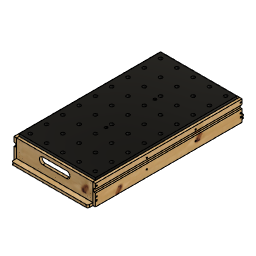
Make_Werkbank v11 (Autodesk Fusion 360 design; units mm, degrees)
Autodesk Fusion 360 part; units mm, degrees
note: some values were not read from the file. Set by a fixed rule: which face or edge a step refers to.
sketch "Seite_L" plane through (0, 0, 0) normal (1, 0, 0) x (0, 1, 0)
  line L0 (432, 60) -> (-432, 60)
  line L1 (-432, 60) -> (-432, -60)
  line L2 (-432, -60) -> (432, -60)
  line L3 (432, -60) -> (432, 60)
  line L4 (432, 60) -> (-432, -60) construction
  line L5 (-432, 60) -> (432, -60) construction
  line L6 (432, 30) -> (-432, 30)
  line L7 (-432, 30) -> (-432, 10)
  line L8 (-432, 10) -> (432, 10)
  line L9 (432, 10) -> (432, 30)
  line L10 (-424.5, -60) -> (-424.5, 60) construction
  line L11 (424.5, -60) -> (424.5, 60) construction
  circle A0 centre (-424.5, 45) radius 4
  circle A1 centre (-424.5, -30) radius 4
  circle A2 centre (-424.5, -10) radius 4
  line L12 (0, -60) -> (0, 60) construction
  circle A3 centre (424.5, 45) radius 4
  circle A4 centre (424.5, -30) radius 4
  circle A5 centre (424.5, -10) radius 4
  point P0 (424.5, 60)
  dimension "d10" = 864
  dimension "d11" = 120
  dimension "d58" = 864
  dimension "d59" = 20
  dimension "d65" = 30
  dimension "d67" = 7.5
  dimension "d68" = 7.5
  dimension "d70" = 8
  dimension "d71" = 15
  dimension "d72" = 8
  dimension "d73" = 8
  dimension "d74" = 30
  dimension "d75" = 20
  constraint horizontal L0
  constraint perpendicular L0 L1
  constraint parallel L1 L3
  constraint coincident L4 origin
  constraint coincident L5 origin
  constraint horizontal L6
  constraint vertical L7
  constraint horizontal L8
  constraint vertical L9
  constraint coincident L3 L6.start
  constraint coincident L2 L10.start
  constraint coincident L0 L10.end
  constraint perpendicular L0 L10
  constraint coincident L2 L11.start
  constraint coincident L0 P0
  constraint perpendicular L0 L11
  constraint coincident L10 A0.centre
  constraint coincident L10 A1.centre
  constraint coincident L10 A2.centre
  constraint midpoint L2 L12.start
  constraint midpoint L0 L12.end
  constraint symmetric L10.end L12 P0
  constraint symmetric A0 L12 A3
  constraint symmetric A1 L12 A4
  constraint symmetric A2 L12 A5
  measures "d10" distance of L1.end L2.end
  measures "d11" distance of L0.end L1.end
  measures "d58" distance of L6.start L6.end
  measures "d59" distance of L6.start L8.end
  measures "d65" distance of L0 L6
  measures "d67" distance of L1 L10
  measures "d68" distance of L3 L11
  measures "d70" diameter of A0
  measures "d71" distance of L0 A0.centre
  measures "d72" diameter of A1
  measures "d73" diameter of A2
  measures "d74" distance of L2 A1.centre
  measures "d75" distance of A1.centre A2.centre
extrude "Extrude1" add sketch "Seite_L" along normal blind 15 contours L0 L1 L3 L6 | L1 L3 L6 L7 L8 L9 | L1 L2 L3 L8 | A0 | A1 | A2 | A3 | A4 | A5 makes body 1
copy_body "CopyPasteBodies2" bodies 1 makes body 2
move_body "Move2" bodies 2 to x (1, 0, 0) y (0, 1, 0) z (0, 0, 1) at (465, 0, 0)
sketch "Seite_K" plane through (0, 0, 0) normal (0, 1, 0) x (1, 0, 0)
  line L0 (15, 45) -> (465, 45)
  line L1 (465, 45) -> (465, -60)
  line L2 (465, -60) -> (15, -60)
  line L3 (15, -60) -> (15, 45)
  line L4 (15, 45) -> (465, 45)
  line L5 (465, 45) -> (465, -55)
  line L6 (465, -55) -> (15, -55)
  line L7 (15, -55) -> (15, 45)
  line L8 (240, -55) -> (240, 45) construction
  line L9 (310, 0) -> (170, 0)
  arc A0 (170, 0) -> (170, -40) centre (170, -20) ccw
  line L10 (170, -40) -> (310, -40)
  arc A1 (310, -40) -> (310, 0) centre (310, -20) ccw
  line L11 (310, -20) -> (170, -20) construction
  line L12 (465, -55) -> (15, -55)
  line L13 (15, -55) -> (15, -40)
  line L14 (15, -40) -> (465, -40)
  line L15 (465, -40) -> (465, -55)
  line L16 (465, -47.5) -> (15, -47.5) construction
  circle A2 centre (432, -47.5) radius 4
  circle A3 centre (336, -47.5) radius 4
  circle A4 centre (240, -47.5) radius 4
  circle A5 centre (144, -47.5) radius 4
  circle A6 centre (48, -47.5) radius 4
  line L17 (465, -60) -> (15, -60)
  line L18 (15, -60) -> (15, -79) construction
  line L19 (15, -79) -> (465, -79) construction
  line L20 (465, -79) -> (465, -60) construction
  circle A7 centre (240, -22) radius 6
  point P0 (240, -20)
  dimension "d16" = 450
  dimension "d17" = 105
  dimension "d28" = 100
  dimension "d54" = 70
  dimension "d55" = 40
  dimension "d96" = 450
  dimension "d97" = 15
  dimension "d98" = 8
  dimension "d99" = 33
  dimension "d103" = 0
  dimension "d144" = 450
  dimension "d145" = 19
  dimension "d146" = 12
  dimension "d155" = 57
  constraint horizontal L0
  constraint vertical L1
  constraint horizontal L2
  constraint vertical L3
  constraint horizontal L4
  constraint vertical L5
  constraint horizontal L6
  constraint vertical L7
  constraint midpoint L6 L8.start
  constraint midpoint L0 L8.end
  constraint perpendicular L0 L8
  constraint tangent L9 A0
  constraint tangent A0 L10
  constraint parallel L9 L10
  constraint tangent L10 A1
  constraint tangent L9 A1
  constraint perpendicular L8 L11
  constraint coincident L8 P0
  constraint midpoint L11 P0
  constraint horizontal L12
  constraint vertical L13
  constraint horizontal L14
  constraint vertical L15
  constraint midpoint L15 L16.start
  constraint midpoint L13 L16.end
  constraint coincident L16 A2.centre
  constraint collinear L10 L14
  constraint horizontal L17
  constraint vertical L18
  constraint horizontal L19
  constraint vertical L20
  constraint coincident L8 A7.centre
  measures "d16" distance of L0.start L0.end
  measures "d17" distance of L0.start L2.end
  measures "d28" distance of L0.start L6.end
  measures "d54" distance of A0.centre P0
  measures "d55" diameter of A0
  measures "d96" distance of L5.end L6.end
  measures "d97" distance of L5.end L14.end
  measures "d98" diameter of A2
  measures "d99" distance of L5 A2.centre
  measures "d144" distance of L1.end L2.end
  measures "d145" distance of L1.end L19.end
  measures "d146" diameter of A7
  measures "d155" distance of L19 A7.centre
extrude "Extrude2" add sketch "Seite_K" against normal blind 15 from surface at 432 separate body contours L0 L1 L3 L4 L5 L7 L9 A0 A1 L14 | L1 L3 L5 L6 L7 L10 L12 L13 L14 L15 | L1 L2 L3 L6 L12 L17 | A2 | A3 | A4 | A5 | A6 makes body 3
copy_body "CopyPasteBodies3" bodies 3 makes body 4
move_body "Move3" bodies 4 to x (1, 0, 0) y (0, 1, 0) z (0, 0, 1) at (0, -849, 0)
sketch "Top" plane through (0, 0, 60) normal (0, 0, 1) x (-1, 0, 0)
  line L0 (-465, 417) -> (-15, 417)
  line L1 (-15, 417) -> (-15, 432)
  line L2 (-15, 432) -> (-465, 432)
  line L3 (-465, 432) -> (-465, 417)
  line L4 (-465, 417) -> (-15, 417)
  line L5 (-15, 417) -> (-15, -417)
  line L6 (-15, -417) -> (-465, -417)
  line L7 (-465, -417) -> (-465, 417)
  line L8 (-15, 417) -> (-465, 417)
  line L9 (-465, 417) -> (-465, 432)
  line L10 (-465, 432) -> (-15, 432)
  line L11 (-15, 432) -> (-15, 417)
  line L12 (-15, 424.5) -> (-465, 424.5) construction
  circle A0 centre (-48, 424.5) radius 4
  line L13 (0, 432) -> (0, -432)
  circle A1 centre (-144, 424.5) radius 4
  circle A2 centre (-240, 424.5) radius 4
  circle A3 centre (-336, 424.5) radius 4
  circle A4 centre (-432, 424.5) radius 4
  line L14 (-15, 0) -> (-465, 0) construction
  circle A5 centre (-336, -424.5) radius 4
  circle A6 centre (-144, -424.5) radius 4
  circle A7 centre (-48, -424.5) radius 4
  circle A8 centre (-240, -424.5) radius 4
  circle A9 centre (-432, -424.5) radius 4
  line L15 (-465, 129) -> (-15, 129) construction
  line L16 (-465, -159) -> (-465.0582, -159)
  line L17 (-465.0582, -159) -> (-15, -159) construction
  circle A10 centre (-240, 129) radius 4
  circle A11 centre (-240, 129) radius 8
  circle A12 centre (-240.0291, -159) radius 4
  circle A13 centre (-240.0291, -159) radius 8
  line L18 (-240, 417) -> (-240, -417) construction
  dimension "d24" = 450
  dimension "d25" = 834
  dimension "d83" = 8
  dimension "d84" = 48
  dimension "d88" = 0
  dimension "d134" = 288
  dimension "d135" = 288
  dimension "d136" = 8
  dimension "d141" = 16
  dimension "d142" = 8
  dimension "d143" = 16
  constraint horizontal L4
  constraint vertical L5
  constraint horizontal L6
  constraint vertical L7
  constraint coincident L0.start L3.end
  constraint horizontal L8
  constraint vertical L9
  constraint horizontal L10
  constraint vertical L11
  constraint coincident L2.end L3.start
  constraint coincident L0.end L1.start
  constraint midpoint L11 L12.start
  constraint midpoint L9 L12.end
  constraint coincident L12 A0.centre
  constraint midpoint L5 L14.start
  constraint midpoint L7 L14.end
  constraint symmetric A0 L14 A7
  constraint symmetric A1 L14 A6
  constraint symmetric A2 L14 A8
  constraint symmetric A3 L14 A5
  constraint symmetric A4 L14 A9
  constraint coincident L7 L15.start
  constraint coincident L5 L15.end
  constraint perpendicular L5 L15
  constraint coincident L7 L16.start
  constraint perpendicular L7 L16
  constraint coincident L5 L17.end
  constraint perpendicular L5 L17
  constraint midpoint L15 A10.centre
  constraint concentric A10 A11
  constraint midpoint L17 A12.centre
  constraint concentric A12 A13
  constraint midpoint L8 L18.start
  constraint midpoint L6 L18.end
  measures "d24" distance of L0.start L0.end
  measures "d25" distance of L0.start L6.end
  measures "d83" diameter of A0
  measures "d84" distance of A0.centre L13
  measures "d134" distance of L4 L15
  measures "d135" distance of L15 L17
  measures "d136" diameter of A10
  measures "d141" diameter of A11
  measures "d142" diameter of A12
  measures "d143" diameter of A13
extrude "Extrude3" add sketch "Top" along normal blind 19 separate body contours L0 L4 L5 L6 L7 L8 | A10 | A11 | A12 | A13 makes body 5
extrude "Extrude4" add sketch "Seite_K" along normal blind 15 from surface at 151.5 separate body contours L0 L1 L3 L4 L5 L7 L9 A0 A1 L14 | L1 L3 L5 L6 L7 L10 L12 L13 L14 L15 | L9 A0 L10 A1 L14 | A2 | A3 | A4 | A5 | A6 | A7 makes body 6
copy_body "CopyPasteBodies4" bodies 6 makes body 7
move_body "Move4" bodies 7 to x (1, 0, 0) y (0, 1, 0) z (0, 0, 1) at (0, -288, 0)
move_body "Align1" bodies 5 to x (1, 0, 0) y (0, 1, 0) z (0, 0, 1) at (0, 0, -5)
sketch "Fuss" plane through (0, 0, -45) normal (0, 0, -1) x (1, 0, 0)
  line L0 (15, 417) -> (465, 417)
  line L1 (465, 417) -> (465, 432)
  line L2 (465, 432) -> (15, 432)
  line L3 (15, 432) -> (15, 417)
  line L4 (15, 417) -> (465, 417)
  line L5 (465, 417) -> (465, 462)
  line L6 (465, 462) -> (15, 462)
  line L7 (15, 462) -> (15, 417)
  dimension "d32" = 450
  dimension "d33" = 45
  constraint horizontal L4
  constraint vertical L5
  constraint horizontal L6
  constraint vertical L7
  constraint coincident L0.start L3.end
  measures "d32" distance of L0.start L0.end
  measures "d33" distance of L0.start L6.end
extrude "Extrude5" add sketch "Fuss" along normal blind 15 separate body makes body 8
copy_body "CopyPasteBodies5" bodies 8 makes body 9
move_body "Move6" bodies 9 to x (1, 0, 0) y (0, 1, 0) z (0, 0, 1) at (0, 879, 0)
sketch "LochRaster" plane through (0, 0, 74) normal (0, 0, 1) x (-1, 0, 0)
  line L0 (-465, -417) -> (-15, -417)
  line L1 (-15, -417) -> (-15, 417)
  line L2 (-15, 417) -> (-465, 417)
  line L3 (-465, 417) -> (-465, -417)
  circle A0 centre (-432, 384) radius 10
  line L4 (-480, -432) -> (-480, 432)
  line L5 (-465, 432) -> (-15, 432)
  line L6 (0, -432) -> (0, 432)
  circle A1 centre (-336, 384) radius 10
  circle A2 centre (-240, 384) radius 10
  circle A3 centre (-144, 384) radius 10
  circle A4 centre (-48, 384) radius 10
  circle A5 centre (-240, 288) radius 10
  circle A6 centre (-432, 288) radius 10
  circle A7 centre (-48, 288) radius 10
  circle A8 centre (-336, 288) radius 10
  circle A9 centre (-144, 288) radius 10
  circle A10 centre (-240, 192) radius 10
  circle A11 centre (-432, 192) radius 10
  circle A12 centre (-48, 192) radius 10
  circle A13 centre (-336, 192) radius 10
  circle A14 centre (-144, 192) radius 10
  circle A15 centre (-240, 96) radius 10
  circle A16 centre (-432, 96) radius 10
  circle A17 centre (-48, 96) radius 10
  circle A18 centre (-336, 96) radius 10
  circle A19 centre (-144, 96) radius 10
  circle A20 centre (-240, 0) radius 10
  circle A21 centre (-432, 0) radius 10
  circle A22 centre (-48, 0) radius 10
  circle A23 centre (-336, 0) radius 10
  circle A24 centre (-144, 0) radius 10
  circle A25 centre (-240, -96) radius 10
  circle A26 centre (-432, -96) radius 10
  circle A27 centre (-48, -96) radius 10
  circle A28 centre (-336, -96) radius 10
  circle A29 centre (-144, -96) radius 10
  circle A30 centre (-240, -192) radius 10
  circle A31 centre (-432, -192) radius 10
  circle A32 centre (-48, -192) radius 10
  circle A33 centre (-336, -192) radius 10
  circle A34 centre (-144, -192) radius 10
  circle A35 centre (-240, -288) radius 10
  circle A36 centre (-432, -288) radius 10
  circle A37 centre (-48, -288) radius 10
  circle A38 centre (-336, -288) radius 10
  circle A39 centre (-144, -288) radius 10
  circle A40 centre (-240, -384) radius 10
  circle A41 centre (-432, -384) radius 10
  circle A42 centre (-48, -384) radius 10
  circle A43 centre (-336, -384) radius 10
  circle A44 centre (-144, -384) radius 10
  line L7 (-465, -432) -> (-15, -432)
  dimension "d36" = 20
  dimension "d37" = 48
  dimension "d40" = 48
  dimension "d43" = 96
  dimension "d44" = -200
  dimension "d45" = 48
  dimension "d46" = 96
  dimension "d49" = 0
  dimension "d50" = -96
  dimension "d51" = 48
  measures "d36" diameter of A0
  measures "d37" distance of A0.centre L4
  measures "d40" distance of A0.centre L5
  measures "d45" distance of A4.centre L6
  measures "d46" distance of A0.centre A1.centre
  measures "d51" distance of A41.centre L7
extrude "Extrude6" cut sketch "LochRaster" against normal blind 19 contours A0 | A1 | A2 | A3 | A4 | A5 | A6 | A7 | A8 | A9 | A10 | A11 | A12 | A13 | A14 | A15 | A16 | A17 | A18 | A19 | A20 | A21 | A22 | A23 | A24 | A25 | A26 | A27 | A28 | A29 | A30 | A31 | A32 | A33 | A34 | A35 | A36 | A37 | A38 | A39 | A40 | A41 | A42 | A43 | A44 bodies 5
extrude "Extrude7" cut sketch "Seite_L" along normal blind 10 contours L1 L3 L6 L7 L8 L9 bodies 1
extrude "Extrude8" cut sketch "Seite_L" against normal blind 10 from surface at 480 contours L1 L3 L6 L7 L8 L9 bodies 2
extrude "Extrude9" cut sketch "Seite_L" along normal blind 30 contours A0 | A1 | A2 | A3 | A4 | A5 bodies 1 3 4 8 9
extrude "Extrude10" cut sketch "Seite_L" against normal blind 30 from surface at 480 contours A0 | A1 | A2 | A3 | A4 | A5 bodies 2 3 4 8 9
fillet "Fillet1" radius 10 4 edges at (15, -462, -52.5) (465, -462, -52.5) (15, 462, -52.5) (465, 462, -52.5) on bodies 8 9
extrude "Extrude11" cut sketch "Top" along normal blind 30 from surface at -120 contours A0 | A1 | A2 | A3 | A4 bodies 4 8
extrude "Extrude12" cut sketch "Top" along normal blind 30 from surface at -120 contours A5 | A6 | A7 | A8 | A9 bodies 3 9
extrude "Extrude13" add sketch "Seite_K" along normal blind 15 from surface at -417 separate body contours L1 L3 L5 L6 L7 L10 L12 L13 L14 L15 makes body 10
copy_body "CopyPasteBodies6" bodies 10 makes body 11
move_body "Move7" bodies 11 to x (1, 0, 0) y (0, 1, 0) z (0, 0, 1) at (0, 819, 0)
extrude "Extrude14" cut sketch "Seite_K" against normal blind 7.5 from surface at -417 contours A2 | A3 | A4 | A5 | A6 bodies 4
extrude "Extrude15" cut sketch "Seite_K" along normal blind 7.5 from surface at 417 contours A2 | A3 | A4 | A5 | A6 bodies 3
sketch "StirnStrebe" plane through (15, 0, 0) normal (-1, 0, 0) x (0, -1, 0)
  line L0 (-151.5, -45) -> (-151.5, 55)
  line L1 (-151.5, 55) -> (-166.5, 55)
  line L2 (-166.5, 55) -> (-166.5, -45)
  line L3 (-166.5, -45) -> (-151.5, -45)
  line L4 (-159, 55) -> (-159, -45) construction
  circle A0 centre (-159, 40) radius 4
  circle A1 centre (-159, -20) radius 4
  line L5 (0, 0) -> (0, 5.9408)
  line L6 (0, 5.9408) -> (0, 120) construction
  dimension "d119" = 8
  dimension "d120" = 8
  dimension "d121" = 25
  dimension "d129" = 15
  constraint midpoint L1 L4.start
  constraint midpoint L3 L4.end
  constraint coincident L4 A0.centre
  constraint coincident L4 A1.centre
  constraint coincident L5.start origin
  constraint vertical L5
  constraint parallel L5 L6
  measures "d119" diameter of A0
  measures "d120" diameter of A1
  measures "d121" distance of L3 A1.centre
  measures "d129" distance of L1 A0.centre
sketch "StirnStrebe2" plane through (15, 0, 0) normal (-1, 0, 0) x (0, -1, 0)
  line L0 (136.5, -45) -> (136.5, 55)
  line L1 (136.5, 55) -> (121.5, 55)
  line L2 (121.5, 55) -> (121.5, -45)
  line L3 (121.5, -45) -> (136.5, -45)
  line L4 (129, 55) -> (129, -45) construction
  circle A0 centre (129, 40) radius 4
  circle A1 centre (129, -20) radius 4
  dimension "d123" = 8
  dimension "d124" = 8
  dimension "d125" = 25
  dimension "d130" = 15
  constraint midpoint L1 L4.start
  constraint midpoint L3 L4.end
  constraint coincident L4 A0.centre
  constraint coincident L4 A1.centre
  measures "d123" diameter of A0
  measures "d124" diameter of A1
  measures "d125" distance of L3 A1.centre
  measures "d130" distance of L1 A0.centre
extrude "Extrude16" cut sketch "StirnStrebe" sketch "StirnStrebe2" along normal up to surface contours A0 | A1 of sketch 2 contours A0 | A1 end surface through (0, 0, 0) normal (-1, 0, 0) offset 0 bodies 1
extrude "Extrude17" cut sketch "StirnStrebe" sketch "StirnStrebe2" along normal up to surface contours A0 | A1 of sketch 2 contours A0 | A1 start surface through (465, 0, 0) normal (-1, 0, 0) end surface through (480, 0, 0) normal (1, 0, 0) offset 0 bodies 2
extrude "Extrude18" cut sketch "Seite_K" against normal blind 15 from surface at -121.5 contours A7 bodies 7
extrude "Extrude19" cut sketch "Seite_K" along normal blind 15 from surface at 151.5 contours A7 bodies 6
extrude "Extrude20" cut sketch "Top" along normal up to surface (14 mm away) contours A10 | A12 bodies 5
extrude "Extrude21" cut sketch "Top" against normal blind 7 from surface at 14 contours A11 | A13 bodies 5
extrude "Extrude22" cut sketch "Top" against normal blind 41.5 contours A10 | A12 bodies 6 7
copy_body "Body->Comp1" bodies 1 removing the originals makes body 12 in component "Seite_L1"
copy_body "Body->Comp2" bodies 2 removing the originals makes body 13 in component "Seite_L2"
copy_body "Body->Comp3" bodies 3 removing the originals makes body 14 in component "Seite_K1"
copy_body "Body->Comp4" bodies 4 removing the originals makes body 15 in component "Seite_K2"
copy_body "Body->Comp5" bodies 5 removing the originals makes body 16 in component "Platte"
copy_body "Body->Comp6" bodies 6 removing the originals makes body 17 in component "Strebe1"
copy_body "Body->Comp7" bodies 7 removing the originals makes body 18 in component "Strebe2"
copy_body "Body->Comp8" bodies 8 removing the originals makes body 19 in component "Fuss1"
copy_body "Body->Comp9" bodies 9 removing the originals makes body 20 in component "Fuss2"
copy_body "Body->Comp10" bodies 10 removing the originals makes body 21 in component "Auflage1"
copy_body "Body->Comp11" bodies 11 removing the originals makes body 22 in component "Auflage2"
move_body "Move5" [suppressed]
component "Seite_L1" placed x (1, 0, 0) y (0, 1, 0) z (0, 0, 1) at (0, 0, 0)
component "Seite_L2" placed x (1, 0, 0) y (0, 1, 0) z (0, 0, 1) at (0, 0, 0)
component "Seite_K1" placed x (1, 0, 0) y (0, 1, 0) z (0, 0, 1) at (0, 0, 0)
component "Seite_K2" placed x (1, 0, 0) y (0, 1, 0) z (0, 0, 1) at (0, 0, 0)
component "Platte" placed x (1, 0, 0) y (0, 1, 0) z (0, 0, 1) at (0, 0, 0)
component "Strebe1" placed x (1, 0, 0) y (0, 1, 0) z (0, 0, 1) at (0, 0, 0)
component "Strebe2" placed x (1, 0, 0) y (0, 1, 0) z (0, 0, 1) at (0, 0, 0)
component "Fuss1" placed x (1, 0, 0) y (0, 1, 0) z (0, 0, 1) at (0, 0, 0)
component "Fuss2" placed x (1, 0, 0) y (0, 1, 0) z (0, 0, 1) at (0, 0, 0)
component "Auflage1" placed x (1, 0, 0) y (0, 1, 0) z (0, 0, 1) at (0, 0, 0)
component "Auflage2" placed x (1, 0, 0) y (0, 1, 0) z (0, 0, 1) at (0, 0, 0)
equation "SeiteLang_L = 864 mm"
equation "SeiteLang_B = 120 mm"
equation "SeiteKurz_L = 450 mm"
equation "SeiteKurz_B = SeiteLang_B - Multi_D"
equation "Strebe_L = SeiteKurz_L"
equation "Strebe_B = SeiteLang_B - Multi_D - 5 mm"
equation "Fuss_L = Strebe_L"
equation "Fuss_B = Multi_D + 30 mm"
equation "Auflage_L = Strebe_L"
equation "d10 = SeiteLang_L"
equation "d11 = SeiteLang_B"
equation "Multi_D = 15 mm"
equation "MDF_D = 19 mm"
equation "d14 = Multi_D"
equation "d16 = SeiteKurz_L"
equation "d17 = SeiteKurz_B"
equation "d19 = -Multi_D"
equation "Platte_L = SeiteLang_L - 2 * Multi_D"
equation "PLatte_B = SeiteKurz_L"
equation "Platte_D = MDF_D"
equation "d24 = PLatte_B"
equation "d25 = Platte_L"
equation "d26 = Platte_D"
equation "d28 = Strebe_B"
equation "d29 = SeiteLang_L / 6 + ( Multi_D / 2 )"
equation "d30 = Multi_D"
equation "d32 = Fuss_L"
equation "d33 = Fuss_B"
equation "d34 = Multi_D"
equation "d36 = LochDurchmesser"
equation "d37 = LochAbstand / 2"
equation "LochAbstand = 96 mm"
equation "LochDurchmesser = 20 mm"
equation "d40 = LochAbstand / 2"
equation "d52 = -MDF_D"
equation "NutSchiene_B = 20 mm"
equation "NutSchiene_T = 10 mm"
equation "d59 = NutSchiene_B"
equation "d60 = NutSchiene_T"
equation "d63 = -NutSchiene_T"
equation "d65 = NutschieneDistFromTop"
equation "NutschieneDistFromTop = 30 mm"
equation "d67 = Multi_D / 2"
equation "d68 = d67"
equation "DübelDicke = 8 mm"
equation "d70 = DübelDicke"
equation "d71 = d65 / 2"
equation "d72 = DübelDicke"
equation "d73 = DübelDicke"
equation "d74 = Multi_D * 2"
equation "d75 = ( d11 - d65 - d74 - NutSchiene_B ) / 2"
equation "d76 = Multi_D * 2"
equation "d79 = -Multi_D * 2"
equation "d83 = DübelDicke"
equation "d84 = LochAbstand / 2"
equation "d87 = -LochAbstand"
equation "d89 = Multi_D * 2"
equation "d93 = Multi_D * 2"
equation "Auflage_B = Multi_D"
equation "d96 = Auflage_L"
equation "d97 = Auflage_B"
equation "d98 = DübelDicke"
equation "d99 = LochAbstand / 2 - Multi_D"
equation "d102 = -LochAbstand"
equation "d105 = Multi_D"
equation "d108 = -Multi_D / 2"
equation "d111 = Multi_D / 2"
equation "d119 = DübelDicke"
equation "d120 = DübelDicke"
equation "d121 = Strebe_B / 4"
equation "d123 = DübelDicke"
equation "d124 = DübelDicke"
equation "d125 = Strebe_B / 4"
equation "d129 = NutschieneDistFromTop / 2"
equation "d130 = NutschieneDistFromTop / 2"
equation "d134 = SeiteLang_L / 3"
equation "d135 = d134"
equation "d136 = M8_Körper"
equation "ZylinderMutterDurch = 12 mm"
equation "M8_Körper = 8 mm"
equation "M8_Kopf_D = 16 mm"
equation "M8_Kopf_H = 7 mm"
equation "d141 = M8_Kopf_D"
equation "d142 = M8_Körper"
equation "d143 = M8_Kopf_D"
equation "d144 = SeiteKurz_L"
equation "d145 = MDF_D"
equation "d146 = ZylinderMutterDurch"
equation "M8_LängeTotal = 51 mm"
equation "d150 = -Multi_D"
equation "d153 = Multi_D"
equation "d155 = M8_LängeTotal + ZylinderMutterDurch / 2"
equation "d159 = -M8_Kopf_H"
equation "d161 = -M8_LängeTotal + MDF_D / 2"
named bodies: "Seite_L1", "Seite_L2", "Seite_K1", "Seite_K2", "Platte", "Strebe1", "Strebe2", "Fuss1", "Fuss2", "Auflage1", "Auflage", "Auflage2"
